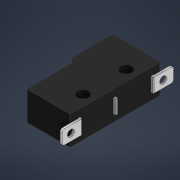
# Autodesk Inventor part: Glicky_3D
Saved by Autodesk Inventor 2022.1 (Build 261234000, 234)
## iProperties
Created: 2021-11-02
Part Number: Glicky_3D
Material: Generisch
Document SubType Name: Modeling
Designer: Rama
Density: 1 g/cm^3
Appearance: Vorgabe
Author: Rama
Autodesk Inventor part; units mm, degrees
ref_plane "YZ Plane" through (0, 0, 0) normal (1, 0, 0) x (0, 1, 0)
ref_plane "XZ Plane" through (0, 0, 0) normal (0, 1, 0) x (-1, 0, 0)
ref_plane "XY Plane" through (0, 0, 0) normal (0, 0, 1) x (1, 0, 0)
sketch "Skizze1" plane through (0, 0, 0) normal (0, 1, 0) x (-1, 0, 0)
  line L0 (5, 10) -> (-5, 10)
  line L1 (-5, 10) -> (-5, -10)
  line L2 (-5, -10) -> (5, -10)
  line L3 (5, -10) -> (5, 10)
  line L4 (5, 10) -> (-5, -10) construction
  line L5 (-5, 10) -> (5, -10) construction
  line L6 (5, -10) -> (6, -10)
  line L7 (6, -10) -> (6, 0)
  line L8 (6, 0) -> (5, 0)
  line L9 (5, 0) -> (5, -10)
  point P0 (0, 0)
  dimension "d0" = 10
  dimension "d1" = 20
  dimension "d2" = 1
  constraints: 20 end point, 4 parallel, 2 horizontal, 2 midpoint, 2 perpendicular
  measures "d0" distance of L2.end L1.end
  measures "d1" distance of L1.end L0.end
  measures "d2" distance of L8.end L7.end
extrude "Extrusion1" add sketch "Skizze1" along normal blind 6.35
sketch "Skizze2" plane through (-6, 0, -10) normal (-1, 0, 0) x (0, 0, 1)
  line L0 (0, 0) -> (0, 6.35) projected
  line L1 (0, 0) -> (10, 0) projected
  line L2 (0, 6.35) -> (8.15, 6.35)
  line L3 (8.15, 6.35) -> (8.15, 0)
  line L4 (8.15, 0) -> (0, 0)
  line L5 (0, 0) -> (0, 6.35)
  line L6 (8.15, 6.35) -> (6.15, 6.35)
  line L7 (6.15, 6.35) -> (6.15, 0)
  line L8 (6.15, 0) -> (8.15, 0)
  line L9 (8.15, 0) -> (8.15, 6.35)
  line L10 (6.15, 4.89) -> (8.15, 4.89)
  line L11 (8.15, 4.89) -> (8.15, 1.46)
  line L12 (8.15, 1.46) -> (6.15, 1.46)
  line L13 (6.15, 1.46) -> (6.15, 4.89)
  line L14 (6.15, 4.89) -> (8.15, 1.46) construction
  line L15 (8.15, 4.89) -> (6.15, 1.46) construction
  point P0 (7.15, 3.175)
  point P1 (8.15, 1.46)
  dimension "d5" = 8.15
  dimension "d6" = 2
  dimension "d7" = 2
  dimension "d8" = 3.43
  constraints: 28 end point, 6 parallel, 3 horizontal, 3 perpendicular, 2 midpoint, 2 point on line
  measures "d5" distance of L3.end L4.end
  measures "d6" distance of L8.end L7.end
  measures "d7" distance of L11.end L12.end
  measures "d8" distance of L10.end L11.end
extrude "Extrusion2" add sketch "Skizze2" along normal blind 1.15 contours L7 L10 L3 L12
sketch "Skizze3" plane through (-6, 4.89, -1.85) normal (0, 1, 0) x (1, 0, 0)
  line L0 (0, 2) -> (0, 0) projected
  line L1 (0, 2) -> (-1.15, 2) projected
  line L2 (-1.15, 0) -> (-1.15, 2) projected
  line L3 (0, 0) -> (-1.15, 0) projected
  circle A0 centre (1.35, 1) radius 2.5
  point P0 (6, -1.85)
  point P1 (-1.15, 1)
  point P2 (-0.9413, 0)
  point P3 (-0.9413, 2)
  dimension "d11" = 5
  constraints: 1 midpoint, 3 other
extrude "Extrusion3" cut sketch "Skizze3" against normal through all contours A0 L2 L1 | L3 L2 A0
fillet "Rundung1" radius 0.2 2 edges at (-6.9413, 3.175, -1.85) (-6.9413, 3.175, -3.85)
chamfer "Fase1" distance 1 angle 45 1 edges at (-6, 3.175, 0)
fillet "Rundung2" radius 0.2 4 edges at (-5, 3.175, 10) (5, 3.175, 10) (5, 3.175, -10) (-6, 3.175, -10)
move faces "Verschieben1" translate (-0.4, 0, 0) faces at (4.8149, 2.1167, 9.9994) (4.936, 2.1167, -9.9466) (5, 2.1167, 3.2667)
sketch "Skizze4" plane through (4.6, 0, 9.8) normal (1, 0, 0) x (0, 0, -1)
  line L0 (19.6, 6.35) -> (19.6, 0) projected
  line L1 (0, 6.35) -> (19.6, 6.35) projected
  line L2 (0, 0) -> (0, 6.35) projected
  line L3 (0, 0) -> (19.6, 0) projected
  line L4 (1.95, 4.725) -> (17.65, 4.725)
  line L5 (17.65, 4.725) -> (17.65, 1.625)
  line L6 (17.65, 1.625) -> (1.95, 1.625)
  line L7 (1.95, 1.625) -> (1.95, 4.725)
  line L8 (9.8, 0) -> (9.8, 6.35) projected
  line L9 (1.95, 4.725) -> (17.65, 1.625) construction
  line L10 (17.65, 4.725) -> (1.95, 1.625) construction
  line L11 (1.5, 4.725) -> (18.1, 4.725)
  line L12 (18.1, 4.725) -> (18.1, 1.625)
  line L13 (18.1, 1.625) -> (1.5, 1.625)
  line L14 (1.5, 1.625) -> (1.5, 4.725)
  line L15 (1.5, 4.725) -> (18.1, 1.625) construction
  line L16 (18.1, 4.725) -> (1.5, 1.625) construction
  line L17 (9.8, 4.725) -> (9.35, 4.725)
  line L18 (9.35, 4.725) -> (9.35, 1.625)
  line L19 (9.35, 1.625) -> (9.8, 1.625)
  line L20 (9.8, 1.625) -> (9.8, 4.725)
  point P0 (9.8, 3.175)
  point P1 (9.8, 3.175)
  point P2 (17.65, 4.725)
  point P3 (17.65, 1.625)
  point P4 (9.35, 4.725)
  point P5 (9.8, 1.625)
  point P6 (9.8, 4.725)
  point P7 (1.95, 1.625)
  point P8 (1.95, 4.725)
  dimension "d22" = 15.7
  dimension "d23" = 3.1
  dimension "d24" = 16.6
  dimension "d25" = 0.45
  constraints: 32 end point, 7 midpoint, 6 parallel, 3 horizontal, 3 perpendicular, 2 point on line
  measures "d22" distance of L5.end L6.end
  measures "d23" distance of L4.end L5.end
  measures "d24" distance of L12.end L13.end
  measures "d25" distance of L19.end L18.end
extrude "Extrusion4" add sketch "Skizze4" along normal blind 0.55 contours L8 L6 L18 L4 | L11 L12 L13 L5 | L7 L13 L14 L11
sketch "Skizze5" plane through (4.6, 4.725, 8.3) normal (0, 1, 0) x (1, 0, 0)
  line L0 (0, 0) -> (0, 0.45) projected
  line L1 (0, 0) -> (0.55, 0) projected
  line L2 (0.55, 0.45) -> (0.55, 0) projected
  line L3 (0, 0.45) -> (0.55, 0.45) projected
  line L4 (0, 16.15) -> (0, 16.6) projected
  line L5 (0, 16.15) -> (0.55, 16.15) projected
  line L6 (0.55, 16.6) -> (0.55, 16.15) projected
  line L7 (0, 16.6) -> (0.55, 16.6) projected
  line L8 (1, -4.015) -> (0.1, -4.015)
  line L9 (0.1, -4.015) -> (0.1, 20.615)
  line L10 (0.1, 20.615) -> (1, 20.615)
  line L11 (1, 20.615) -> (1, -4.015)
  line L12 (0.55, 7.85) -> (0.55, 8.3) projected
  line L13 (1, -4.015) -> (0.1, 20.615) construction
  line L14 (0.1, -4.015) -> (1, 20.615) construction
  line L15 (0.55, 20.615) -> (0.55, -4.015)
  point P0 (-4.6, 8.3)
  point P1 (0.1, 16.6)
  point P2 (0.1, 0)
  dimension "d28" = 0.9
  dimension "d29" = 24.63
  constraints: 14 end point, 4 midpoint, 2 parallel, 1 horizontal, 1 perpendicular
  measures "d28" distance of L9.end L10.end
  measures "d29" distance of L8.end L9.end
extrude "Extrusion5" add sketch "Skizze5" against normal up to surface (3.1 mm away) contours L1 L15 L8 L9 | L9 L10 L15 L7
fillet "Rundung3" radius 0.2 2 edges at (5.15, 3.175, -7.85) (5.15, 3.175, 7.85)
fillet "Rundung4" radius 0.1 2 edges at (4.7, 3.175, -8.3) (4.7, 3.175, 8.3)
fillet "Rundung5" radius 0.1 2 edges at (5.15, 3.175, 0.45) (5.15, 3.175, 0)
sketch "Skizze6" plane through (5.15, 0, 9.8) normal (1, 0, 0) x (0, 0, -1)
  line L0 (1.75, 4.725) -> (1.75, 1.625) projected
  line L1 (1.75, 4.725) -> (-2.515, 4.725) projected
  line L2 (-2.515, 4.725) -> (-2.515, 1.625) projected
  line L3 (-2.515, 1.625) -> (1.75, 1.625) projected
  line L4 (17.85, 1.625) -> (17.85, 4.725) projected
  line L5 (17.85, 1.625) -> (22.115, 1.625) projected
  line L6 (22.115, 4.725) -> (22.115, 1.625) projected
  line L7 (17.85, 4.725) -> (22.115, 4.725) projected
  circle A0 centre (-0.5825, 3.175) radius 0.75
  circle A1 centre (19.7825, 3.175) radius 0.75
  point P0 (9.8, 0)
  dimension "d35" = 1.5
  dimension "d36" = 1.5
  constraints: 2 centre point
  measures "d35" diameter of A0
  measures "d36" diameter of A1
extrude "Extrusion6" cut sketch "Skizze6" against normal up to surface (0.45 mm away) contours A0 | A1
sketch "Skizze7" plane through (0, 6.35, 0) normal (0, 1, 0) x (1, 0, 0)
  line L0 (3.45, 6) -> (0.95, 6)
  line L1 (0.95, 6) -> (0.95, -6)
  line L2 (0.95, -6) -> (3.45, -6)
  line L3 (3.45, -6) -> (3.45, 6)
  line L4 (3.45, 6) -> (0.95, -6) construction
  line L5 (0.95, 6) -> (3.45, -6) construction
  line L6 (3.45, 3.5) -> (0.95, 3.5)
  line L7 (0.95, 3.5) -> (0.95, -3.5)
  line L8 (0.95, -3.5) -> (3.45, -3.5)
  line L9 (3.45, -3.5) -> (3.45, 3.5)
  line L10 (3.45, 3.5) -> (0.95, -3.5) construction
  line L11 (0.95, 3.5) -> (3.45, -3.5) construction
  circle A0 centre (2.2, 4.75) radius 1.25
  circle A1 centre (2.2, -4.75) radius 1.25
  arc A2 (4.95, 7.85) -> (5.15, 8.05) centre (4.95, 8.05) ccw projected
  line L12 (5.15, 8.05) -> (5.15, 12.315) projected
  line L13 (5.15, 12.315) -> (4.7, 12.315) projected
  line L14 (4.7, 12.315) -> (4.7, 8.4) projected
  arc A3 (4.6, 8.3) -> (4.7, 8.4) centre (4.6, 8.4) ccw projected
  line L15 (4.6, 7.85) -> (4.6, 8.3) projected
  line L16 (4.6, 7.85) -> (4.95, 7.85) projected
  arc A4 (5.15, -8.05) -> (4.95, -7.85) centre (4.95, -8.05) ccw projected
  line L17 (4.6, -7.85) -> (4.95, -7.85) projected
  line L18 (4.6, -8.3) -> (4.6, -7.85) projected
  arc A5 (4.7, -8.4) -> (4.6, -8.3) centre (4.6, -8.4) ccw projected
  line L19 (4.7, -8.4) -> (4.7, -12.315) projected
  line L20 (4.7, -12.315) -> (5.15, -12.315) projected
  line L21 (5.15, -8.05) -> (5.15, -12.315) projected
  point P0 (0, 0)
  point P1 (2.2, 0)
  point P2 (2.2, 0)
  point P3 (2.2, 3.5)
  point P4 (2.2, 6)
  point P5 (2.2, 0)
  dimension "d39" = 2.5
  dimension "d40" = 12
  dimension "d41" = 2.5
  dimension "d42" = 7
  dimension "d43" = 1.7
  dimension "d44" = 24.63
  dimension "d45" = 12.315
  dimension "d46" = 2.95
  constraints: 24 end point, 8 midpoint, 4 parallel, 4 tangent, 2 centre point, 2 horizontal, 2 perpendicular, 2 point on circle
  measures "d39" distance of L2.end L1.end
  measures "d40" distance of L1.end L0.end
  measures "d41" distance of L8.end L7.end
  measures "d42" distance of L7.end L6.end
  measures "d43" distance between parallel lines of L9 L12
  measures "d44" distance between parallel lines of L20 L13
  measures "d45" distance from line of L13 point (2.2, 0)
  measures "d46" distance from line of L12 A0.centre
extrude "Extrusion7" cut sketch "Skizze7" against normal through all contours A0 | A1
fillet "Rundung6" radius 0.6 4 edges at (4.925, 4.725, 12.315) (4.925, 1.625, 12.315) (4.925, 4.725, -12.315) (4.925, 1.625, -12.315)
equation "\"d45\" = 0.5 * d44"
